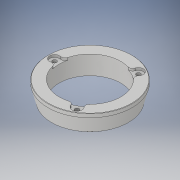
# Autodesk Inventor part: Flywheel Mass
Saved by Autodesk Inventor 2019.4 (Build 234330000, 330)
## iProperties
Created: 2020-02-21
Part Number: Flywheel Mass
Material: Generic
Document SubType Name: Modeling
Designer: admin
Density: 1 g/cm^3
Appearance: Default
Author: admin
Autodesk Inventor part; units mm, degrees
ref_plane "YZ Plane" through (0, 0, 0) normal (1, 0, 0) x (0, 1, 0)
ref_plane "XZ Plane" through (0, 0, 0) normal (0, 1, 0) x (-1, 0, 0)
ref_plane "XY Plane" through (0, 0, 0) normal (0, 0, 1) x (1, 0, 0)
sketch "Sketch1" plane through (0, 0, 0) normal (1, 0, 0) x (0, 1, 0)
  line L0 (0, 41.03) -> (25, 41.03)
  line L1 (25, 41.03) -> (25, 55.88)
  line L2 (25, 55.88) -> (20, 55.88)
  line L3 (20, 55.88) -> (0, 50.88)
  line L4 (0, 50.88) -> (0, 41.03)
  line L5 (0, 0) -> (26.8378, 0) construction
  dimension "d0" = 55.88
  dimension "d1" = 5
  dimension "d2" = 25
  dimension "d3" = 20
  dimension "d4" = 41.03
  constraints: 12 end point, 2 horizontal, 2 perpendicular, 1 parallel, 1 point on line
  measures "d0" distance from line of L5.start L2
  measures "d1" vertical distance of L2.end L3.end
  measures "d2" distance of L0.start L0.end
  measures "d3" horizontal distance of L2.end L3.end
  measures "d4" distance from line of L5.start L0
revolve "Revolution1" add sketch "Sketch1" angle 360 about axis through (0, 0, 0) along (0, 1, 0)
sketch "Sketch2" plane through (0, 25, 0) normal (0, 1, 0) x (1, 0, 0)
  circle A0 centre (-47.18, 0) radius 6.65
  circle A1 centre (-47.18, 0) radius 2.75
  line L0 (-47.18, 0) -> (0, 0) construction
  dimension "d6" = 13.3
  dimension "d7" = 5.5
  dimension "d8" = 47.18
  constraints: 2 centre point, 2 end point, 1 coincident, 1 horizontal
  measures "d6" diameter of A0
  measures "d7" diameter of A1
  measures "d8" distance of L0.start L0.end
extrude "Extrusion1" cut sketch "Sketch2" against normal blind 3.1 contours A0 | A1
fillet "Fillet1" radius 5 2 edges at (-40.9622, 23.45, 2.3582) (-40.9622, 23.45, -2.3582)
sketch "Sketch3" plane through (0, 21.9, 0) normal (0, 1, 0) x (1, 0, 0)
  arc A0 (-45.7105, 6.4856) -> (-45.7105, -6.4856) centre (-47.18, 0) ccw projected
  point P0 (0, 0)
  constraints: 1 coincident
hole "Hole1" at (-47.18, 21.9, 0) direction (0, -1, 0) diameter 5.5 end through all
chamfer "Chamfer1" distance 0.5 angle 45 2 edges at (0, 0, -50.88) (0, 25, -55.88)
pattern_circular "Circular Pattern1" count 3 over 360 about axis through (0, 12.5, 0) along (0, 1, 0) of "Extrusion1", "Hole1", "Fillet1"
body "Solid1"
